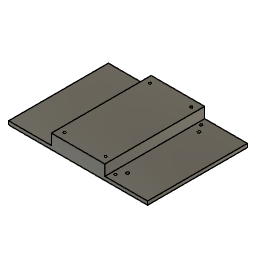
Platform_Riser_V4 (Autodesk Fusion 360 design; units mm, degrees)
part number: 2025-10-16-22-08-15-071
Autodesk Fusion 360 part; units mm, degrees
sketch "Sketch1" plane through (0, 0, 0) normal (0, 0, 1) x (1, 0, 0)
  line L0 (0, 0) -> (195, 0)
  line L1 (195, 0) -> (195, 140)
  line L2 (195, 140) -> (0, 140)
  line L3 (0, 140) -> (0, 0)
  line L4 (60, 140) -> (60, 0)
  line L5 (135, 140) -> (135, 0)
  circle A0 centre (68.5, 10) radius 1.7
  circle A1 centre (126.5, 10) radius 1.7
  line L6 (97.5, 0) -> (97.5, 140) construction
  circle A2 centre (68.5, 130) radius 1.7
  circle A3 centre (126.5, 130) radius 1.7
  line L7 (68.5, 130) -> (68.5, 100) construction
  circle A4 centre (68.5, 107) radius 1.7
  line L8 (126.5, 130) -> (126.5, 100) construction
  circle A5 centre (126.5, 107) radius 1.7
  circle A6 centre (48, 120) radius 2
  line L9 (0, 70) -> (195, 70) construction
  circle A7 centre (48, 20) radius 2
  circle A8 centre (147, 120) radius 2
  circle A9 centre (147, 20) radius 2
  line L10 (50, 0) -> (50, 140) construction
  line L11 (145, 0) -> (145, 140) construction
  circle A10 centre (55, 10) radius 1.7
  circle A11 centre (55, 130) radius 1.7
  circle A12 centre (140, 130) radius 1.7
  circle A13 centre (140, 10) radius 1.7
  dimension "d1" = 140
  dimension "d3" = 60
  dimension "d4" = 60
  dimension "d5" = 3.4
  dimension "d6" = 10
  dimension "d7" = 3.4
  dimension "d10" = 58
  dimension "d11" = 3.4
  dimension "d12" = 3.4
  dimension "d13" = 58
  dimension "d14" = 10
  dimension "d23" = 3.4
  dimension "d24" = 23
  dimension "d25" = 3.4
  dimension "d26" = 23
  dimension "d27" = 4
  dimension "d28" = 4
  dimension "d29" = 100
  dimension "d30" = 4
  dimension "d31" = 4
  dimension "d32" = 100
  dimension "d42" = 75
  dimension "d43" = 50
  dimension "d44" = 50
  dimension "d46" = 3.4
  dimension "d47" = 10
  dimension "d48" = 3.4
  dimension "d49" = 10
  dimension "d50" = 3.4
  dimension "d51" = 10
  dimension "d52" = 3.4
  dimension "d53" = 10
  dimension "d54" = 5
  dimension "d55" = 5
  dimension "d56" = 5
  dimension "d57" = 5
  constraint horizontal L0
  constraint vertical L1
  constraint horizontal L2
  constraint vertical L3
  constraint coincident L0.start L3.end
  constraint coincident L2 L4.start
  constraint coincident L0 L4.end
  constraint perpendicular L0 L4
  constraint coincident L2 L5.start
  constraint coincident L0 L5.end
  constraint perpendicular L0 L5
  constraint midpoint L0 L6.start
  constraint midpoint L2 L6.end
  constraint symmetric A0.centre A1.centre L6
  constraint symmetric L6 A2.centre A3.centre
  constraint coincident A2.centre L7.start
  constraint vertical L7
  constraint coincident L7 A4.centre
  constraint coincident A3.centre L8.start
  constraint vertical L8
  constraint coincident L8 A5.centre
  constraint midpoint L3 L9.start
  constraint midpoint L1 L9.end
  constraint symmetric A6.centre L9 A7.centre
  constraint symmetric L9 A8.centre A9.centre
  constraint coincident L0 L10.start
  constraint coincident L2 L10.end
  constraint perpendicular L2 L10
  constraint tangent A7 L10
  constraint coincident L0 L11.start
  constraint coincident L2 L11.end
  constraint perpendicular L2 L11
  constraint tangent A9 L11
  measures "d1" distance of L0.start L2.end
  measures "d3" distance of L3 L4
  measures "d4" distance of L1 L5
  measures "d5" diameter of A0
  measures "d6" distance of L0 A0.centre
  measures "d7" diameter of A1
  measures "d10" distance of A0.centre A1.centre
  measures "d11" diameter of A2
  measures "d12" diameter of A3
  measures "d13" distance of A2.centre A3.centre
  measures "d14" distance of L2 A2.centre
  measures "d23" diameter of A4
  measures "d24" distance of A2.centre A4.centre
  measures "d25" diameter of A5
  measures "d26" distance of A3.centre A5.centre
  measures "d27" diameter of A6
  measures "d28" diameter of A7
  measures "d29" distance of A6.centre A7.centre
  measures "d30" diameter of A8
  measures "d31" diameter of A9
  measures "d32" distance of A8.centre A9.centre
  measures "d42" distance of L4 L5
  measures "d43" distance of L3 L10
  measures "d44" distance of L1 L11
  measures "d46" diameter of A10
  measures "d47" distance of L0 A10.centre
  measures "d48" diameter of A11
  measures "d49" distance of L2 A11.centre
  measures "d50" diameter of A12
  measures "d51" distance of L2 A12.centre
  measures "d52" diameter of A13
  measures "d53" distance of L0 A13.centre
  measures "d54" distance of L5 A13.centre
  measures "d55" distance of L5 A12.centre
  measures "d56" distance of L4 A11.centre
  measures "d57" distance of L4 A10.centre
extrude "Extrude1" add sketch "Sketch1" along normal blind 20 contours L0 L2 L4 L5
extrude "Extrude3" add sketch "Sketch1" along normal blind 5 contours L0 L2 L3 L4 | L0 L1 L2 L5
extrude "Extrude4" add sketch "Sketch1" along normal blind 15 contours A0 | A1
extrude "Extrude5" add sketch "Sketch1" along normal blind 10 from surface at 5 contours A2 | A3
extrude "Extrude6" add sketch "Sketch1" along normal blind 15 from surface at 5 contours A4 | A5
equation "d5 = m3_hole_diameter"
equation "d7 = m3_hole_diameter"
equation "d11 = m3_hole_diameter"
equation "d12 = m3_hole_diameter"
equation "d23 = m3_hole_diameter"
equation "d25 = m3_hole_diameter"
equation "d27 = zip_tie_hole_diameter"
equation "d28 = zip_tie_hole_diameter"
equation "d30 = zip_tie_hole_diameter"
equation "d31 = zip_tie_hole_diameter"
equation "zip_tie_hole_diameter = 4 mm"
equation "m3_hole_diameter = 3.4 mm"
equation "d46 = m3_hole_diameter"
equation "d48 = m3_hole_diameter"
equation "d50 = m3_hole_diameter"
equation "d52 = m3_hole_diameter"
